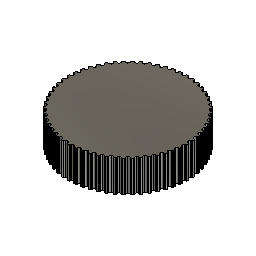
gear_60z (Autodesk Fusion 360 design; units mm, degrees)
Autodesk Fusion 360 part; units mm, degrees
sketch "Sketch1" plane through (0, 0, 0) normal (0, 0, 1) x (1, 0, 0) in component "gt2 pulley"
  circle A0 centre (0, 0) radius 19.0986 construction
  circle A1 centre (0, 0) radius 18.0946 construction
  line L0 (0, 0) -> (0, 19.0986) construction
  line L1 (0, 0) -> (0.9995, 19.0724) construction
  line L2 (0, 0) -> (1.4062, 19.0468) construction
  circle A2 centre (0, 0) radius 18.8446 construction
  arc A3 (0.3914, 18.7061) -> (0.4628, 18.4128) centre (1.3875, 18.7934) ccw
  circle A4 centre (0, 0) radius 18.6946 construction
  arc A5 (0.2438, 18.843) -> (0, 18.8446) centre (0, 0) ccw
  arc A6 (0.3914, 18.7061) -> (0.2438, 18.843) centre (0.2419, 18.693) ccw
  arc A7 (0.4628, 18.4128) -> (0.947, 18.0698) centre (0.976, 18.624) ccw
  arc A8 (0, 18.8446) -> (-0.2438, 18.843) centre (0, 0) ccw
  arc A9 (-0.2438, 18.843) -> (-0.3914, 18.7061) centre (-0.2419, 18.693) ccw
  arc A10 (-0.4628, 18.4128) -> (-0.3914, 18.7061) centre (-1.3875, 18.7934) ccw
  arc A11 (-0.947, 18.0698) -> (-0.4628, 18.4128) centre (-0.976, 18.624) ccw
  arc A12 (0.947, 18.0698) -> (-0.947, 18.0698) centre (0, 0) ccw
  point P0 (1.3875, 18.7934)
  point P1 (0, 18.8446)
  dimension "d18" = 38.1972
  dimension "d19" = 3
  dimension "d22" = 1.004
  dimension "d24" = 0.75
  dimension "d26" = 1
  dimension "d27" = 0.15
  dimension "d28" = 0.15
  dimension "d47" = 0.555
  dimension "d52" = 3.812
  constraint coincident A0.centre A1.centre
  constraint coincident A0 L0.end
  constraint vertical L0
  constraint coincident A0 L1.end
  constraint coincident A0 L2.end
  constraint concentric A1 A2
  constraint coincident A1 A7.end
  constraint coincident L1 A7.end
  constraint coincident A2 P0
  constraint coincident L2 P0
  constraint coincident P0 A3.centre
  constraint coincident A2 P1
  constraint coincident L0 P1
  constraint concentric A2 A4
  constraint coincident P1 A5.end
  constraint coincident A4 A6.centre
  constraint coincident A3.start A6.start
  constraint tangent A3 A6
  constraint tangent A3 A7
  constraint symmetric L0 A7.end A11.start
  constraint symmetric L0 A3.start A9.end
  constraint symmetric L0 A3.end A10.start
  constraint symmetric L0 A3 A10
  constraint symmetric L0 A5.start A8.end
  constraint symmetric L0 P1 A5.end
  constraint symmetric L0 A5 A8
  constraint symmetric L0 A6 A9
  constraint symmetric L0 A7 A11
  constraint coincident A1 A11.start
  constraint tangent A1 A7
  constraint coincident L1 A7.centre
  measures "d18" diameter of A0
  measures "d19" angle of L0 L1
  measures "d22" distance of A0 A1
  measures "d24" distance of A1 A2
  measures "d26" radius of A3
  measures "d27" distance of A2 A4
  measures "d28" radius of A6
  measures "d47" radius of A7
extrude "Extrude1" add sketch "Sketch1" along normal blind 10 makes body 1
pattern_circular "C-Pattern1" count 60 over 360 about axis through (0, 0, 1.75) along (0, 0, 1) of bodies 1 makes body 2 at (-1.9961, 17.9842, 6.6667) makes body 3 at (-3.0384, 17.8377, 3.3333) makes body 4 at (-4.8863, 17.4224, 3.3333) makes body 5 at (-6.6806, 16.8162, 3.3333) makes body 6 at (-9.1383, 15.6175, 6.6667) makes body 7 at (-10.7207, 14.5767, 6.6667) makes body 8 at (-12.1857, 13.3762, 6.6667) makes body 9 at (-13.9287, 11.5501, 6.6667) makes body 10 at (-14.1937, 11.2229, 3.3333) makes body 11 at (-15.289, 9.6778, 3.3333) makes body 12 at (-16.5728, 7.2634, 6.6667) makes body 13 at (-17.2412, 5.4913, 6.6667) makes body 14 at (-17.8377, 3.0384, 6.6667) makes body 15 at (-18.0062, 1.7867, 6.6667) makes body 16 at (-18.0796, 0.7367, 3.3333) makes body 17 at (-18.0576, -1.1572, 3.3333) makes body 18 at (-17.8377, -3.0384, 3.3333) makes body 19 at (-17.4224, -4.8863, 3.3333) makes body 20 at (-16.4871, -7.4558, 6.6667) makes body 21 at (-15.6175, -9.1383, 6.6667) makes body 22 at (-14.5767, -10.7207, 6.6667) makes body 23 at (-13.3762, -12.1857, 6.6667) makes body 24 at (-11.5501, -13.9287, 6.6667) makes body 25 at (-11.2229, -14.1937, 3.3333) makes body 26 at (-8.4018, -16.0257, 6.6667) makes body 27 at (-7.2634, -16.5728, 6.6667) makes body 28 at (-5.4913, -17.2412, 6.6667) makes body 29 at (-3.0384, -17.8377, 6.6667) makes body 30 at (-2.6225, -17.9035, 3.3333) makes body 31 at (-0.7367, -18.0796, 3.3333) makes body 32 at (1.1572, -18.0576, 3.3333) makes body 33 at (3.865, -17.677, 6.6667) makes body 34 at (4.8863, -17.4224, 3.3333) makes body 35 at (6.6806, -16.8162, 3.3333) makes body 36 at (9.1383, -15.6175, 6.6667) makes body 37 at (10.0309, -15.0597, 3.3333) makes body 38 at (12.1857, -13.3762, 6.6667) makes body 39 at (13.9287, -11.5501, 6.6667) makes body 40 at (14.7005, -10.5504, 6.6667) makes body 41 at (15.7228, -8.956, 6.6667) makes body 42 at (16.2169, -8.0266, 3.3333) makes body 43 at (17.2412, -5.4913, 6.6667) makes body 44 at (17.5313, -4.4795, 3.3333) makes body 45 at (17.9035, -2.6225, 3.3333) makes body 46 at (18.0796, -0.7367, 3.3333) makes body 47 at (17.9842, 1.9961, 6.6667) makes body 48 at (17.8377, 3.0384, 3.3333) makes body 49 at (17.1762, 5.6916, 6.6667) makes body 50 at (16.8162, 6.6806, 3.3333) makes body 51 at (15.289, 9.6778, 6.6667) makes body 52 at (15.0597, 10.0309, 3.3333) makes body 53 at (12.9428, 12.6451, 6.6667) makes body 54 at (12.0292, 13.5171, 6.6667) makes body 55 at (10.5504, 14.7005, 6.6667) makes body 56 at (8.956, 15.7228, 6.6667) makes body 57 at (8.0266, 16.2169, 3.3333) makes body 58 at (5.4913, 17.2412, 6.6667) makes body 59 at (4.4795, 17.5313, 3.3333) makes body 60 at (1.7867, 18.0062, 6.6667)
sketch "Sketch2" plane through (0, 0, 10) normal (0, 0, 1) x (-1, 0, 0)
  arc A0 (-9.692, -16.0043) -> (-9.6327, -16.1966) centre (-9.556, -16.0677) ccw
  arc A1 (-9.6327, -16.1966) -> (-9.2104, -16.4404) centre (0, 0) ccw
  arc A2 (-9.2104, -16.4404) -> (-9.0141, -16.3957) centre (-9.137, -16.3096) ccw
  arc A3 (-8.8056, -16.1773) -> (-9.0141, -16.3957) centre (-8.1951, -16.9694) ccw
  arc A4 (-8.2148, -16.1224) -> (-8.8055, -16.1773) centre (-8.4667, -16.6169) ccw
  arc A5 (-9.855, -15.1754) -> (-8.2148, -16.1224) centre (0, 0) ccw
  arc A6 (-9.6072, -15.7145) -> (-9.855, -15.1754) centre (-10.1573, -15.6409) ccw
  arc A7 (-9.692, -16.0043) -> (-9.6072, -15.7145) centre (-10.5984, -15.5818) ccw
  circle A8 centre (0, 0) radius 18.0946
  constraint coincident A1.centre A5.centre
extrude "Extrude2" add sketch "Sketch2" against normal blind 10 contours A5 A8 bodies 1 2 3 4 5 6 7 8 9 10 11 12 13 14 15 16 17 18 19 20 21 22 23 24 25 26 27 28 29 30 31 32 33 34 35 36 37 38 39 40 41 42 43 44 45 46 47 48 49 50 51 52 53 54 55 56 57 58 59 60
extrude "Extrude4" [suppressed] in component "gt2 pulley"
pattern_circular "C-Pattern7" [suppressed] in component "gt2 pulley"
extrude "Extrude3" [suppressed] in component "gt2 pulley"
pattern_circular "C-Pattern6" [suppressed] in component "gt2 pulley"
extrude "Extrude2'" [suppressed] in component "gt2 pulley"
pattern_circular "C-Pattern5" [suppressed] in component "gt2 pulley"
extrude "Extrude1'" [suppressed] in component "gt2 pulley"
pattern_circular "C-Pattern4" [suppressed] in component "gt2 pulley"
pattern_circular "C-Pattern3" [suppressed] in component "gt2 pulley"
pattern_circular "C-Pattern2" [suppressed] in component "gt2 pulley"
pattern_circular "C-Pattern1'" [suppressed] in component "gt2 pulley"
copy_body "Body->Comp1" [suppressed] in component "Component"
copy_body "Body->Comp2" [suppressed] in component "Component'"
copy_body "Body->Comp3" [suppressed] in component "Component''"
copy_body "Body->Comp4" [suppressed] in component "Component'''"
copy_body "Body->Comp5" [suppressed] in component "Component''''"
copy_body "Body->Comp6" [suppressed] in component "Component'''''"
copy_body "Body->Comp7" [suppressed] in component "Component''''''"
copy_body "Body->Comp8" [suppressed] in component "Component'''''''"
copy_body "Body->Comp9" [suppressed] in component "Component''''''''"
copy_body "Body->Comp10" [suppressed] in component "Component'''''''''"
copy_body "Body->Comp11" [suppressed] in component "Component''''''''''"
copy_body "Body->Comp12" [suppressed] in component "Component'''''''''''"
copy_body "Body->Comp13" [suppressed] in component "Component''''''''''''"
copy_body "Body->Comp14" [suppressed] in component "Component'''''''''''''"
copy_body "Body->Comp15" [suppressed] in component "Component''''''''''''''"
copy_body "Body->Comp16" [suppressed] in component "Component'''''''''''''''"
copy_body "Body->Comp17" [suppressed] in component "Component''''''''''''''''"
copy_body "Body->Comp18" [suppressed] in component "Component'''''''''''''''''"
copy_body "Body->Comp19" [suppressed] in component "Component''''''''''''''''''"
copy_body "Body->Comp20" [suppressed] in component "Component'''''''''''''''''''"
component "gt2 pulley" placed x (1, 0, 0) y (0, 1, 0) z (0, 0, 1) at (0, 0, 0)
equation "NumTeeth = 60" comment "min 20"
equation "ToothPitch = 2 mm"
equation "PullyDia = NumTeeth * ToothPitch / PI"
equation "ToothAng = ( ( 360 / NumTeeth ) * 1 deg )"
equation "TransOffsetAngle = ToothAng * 0.2"
equation "Sholulder_Radius = 0.15 mm"
equation "Root_Radius = 0.555 mm"
equation "TransRadius = 1 mm"
equation "ToolHeight = 0.75 mm"
equation "PLD = 0.254 mm"
equation "d18 = PullyDia"
equation "d19 = ToothAng / 2"
equation "d22 = PLD + ToolHeight"
equation "d24 = ToolHeight"
equation "d26 = TransRadius"
equation "d27 = Sholulder_Radius"
equation "d31 = NumTeeth"
equation "d33 = NumTeeth"
equation "d35 = NumTeeth"
equation "d37 = NumTeeth"
equation "d41 = NumTeeth"
equation "d45 = NumTeeth"
equation "d47 = Root_Radius"
equation "d50 = NumTeeth"
